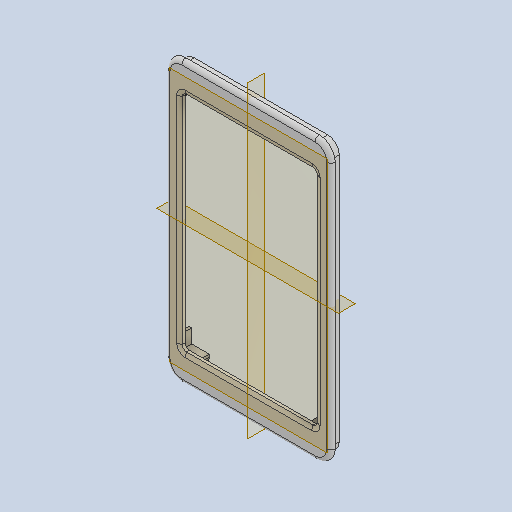
# Autodesk Inventor part: front-bezel
Saved by Autodesk Inventor 2024 (Build 280153000, 153)
## iProperties
Created: 2024-08-25
Part Number: front-bezel
Material: Generic
Document SubType Name: Modeling
Designer: Stefano
Density: 1 g/cm^3
Appearance: Default
Author: Stefano
Autodesk Inventor part; units mm, degrees
ref_plane "YZ Plane" through (0, 0, 0) normal (1, 0, 0) x (0, 1, 0)
ref_plane "Work Plane1" through (0, 0, 2.9972) normal (0, 0, 1) x (1, 0, 0)
ref_plane "Work Plane3" through (-58.9, -99.9, 0) normal (0, 0, 1) x (1, 0, 0)
sketch "Sketch2" plane through (0, 0, 2.9972) normal (0, 0, 1) x (1, 0, 0)
  line L0 (51.1175, 82.55) -> (51.1175, -82.55) construction
  line L1 (-51.1175, 82.55) -> (51.1175, 82.55) construction
  line L2 (-51.1175, -82.55) -> (-51.1175, 82.55) construction
  line L3 (51.1175, -82.55) -> (-51.1175, -82.55) construction
  arc A0 (58.9, 88.5) -> (47.5, 99.9) centre (47.5, 88.5) ccw projected
  line L4 (47.5, 99.9) -> (-47.5, 99.9) projected
  line L5 (58.9, -88.5) -> (58.9, 88.5) projected
  arc A1 (47.5, -99.9) -> (58.9, -88.5) centre (47.5, -88.5) ccw projected
  line L6 (-47.5, -99.9) -> (47.5, -99.9) projected
  arc A2 (-58.9, -88.5) -> (-47.5, -99.9) centre (-47.5, -88.5) ccw projected
  line L7 (-58.9, 88.5) -> (-58.9, -88.5) projected
  arc A3 (-47.5, 99.9) -> (-58.9, 88.5) centre (-47.5, 88.5) ccw projected
  line L8 (48.1175, -79.55) -> (48.1175, 79.55)
  line L9 (48.1175, 79.55) -> (-48.1175, 79.55)
  line L10 (-48.1175, 79.55) -> (-48.1175, -79.55)
  line L11 (-48.1175, -79.55) -> (48.1175, -79.55)
  point P0 (0, 0)
  dimension "d1" = 3
  constraints: 8 end point, 3 other
  measures "d1" distance between parallel lines of L0 L8
extrude "Extrusion1" add sketch "Sketch2" against normal up to surface (2.9972 mm away)
fillet "Fillet1" radius 3 4 edges at (48.1175, 79.55, 1.4986) (48.1175, -79.55, 1.4986) (-48.1175, -79.55, 1.4986) (-48.1175, 79.55, 1.4986)
chamfer "Chamfer1" distance 3 distance2 1 4 edges at (48.1175, 0, 2.9972) (0, -79.55, 2.9972) (-48.1175, 0, 2.9972) (0, 79.55, 2.9972) measured on face at (15.0392, -93.1167, 2.9972)
sketch "Sketch3" plane through (47.5, 99.9, 0) normal (0, 0, -1) x (-1, 0, 0)
  line L0 (98.6175, -17.35) -> (-3.6175, -17.35) construction
  line L1 (98.6175, -182.45) -> (98.6175, -17.35) construction
  line L2 (-3.6175, -182.45) -> (98.6175, -182.45) construction
  line L3 (-3.6175, -17.35) -> (-3.6175, -182.45) construction
  line L4 (95, -196.8) -> (0, -196.8) construction
  arc A0 (-8.4, -188.4) -> (0, -196.8) centre (0, -188.4) ccw construction
  line L5 (-8.4, -188.4) -> (-8.4, -11.4) construction
  arc A1 (0, -3) -> (-8.4, -11.4) centre (0, -11.4) ccw construction
  line L6 (0, -3) -> (95, -3) construction
  arc A2 (103.4, -11.4) -> (95, -3) centre (95, -11.4) ccw construction
  line L7 (103.4, -11.4) -> (103.4, -188.4) construction
  arc A3 (95, -196.8) -> (103.4, -188.4) centre (95, -188.4) ccw construction
  line L8 (-3.7175, -17.25) -> (98.7175, -17.25)
  line L9 (98.7175, -17.25) -> (98.7175, -182.55)
  line L10 (98.7175, -182.55) -> (-3.7175, -182.55)
  line L11 (-3.7175, -182.55) -> (-3.7175, -17.25)
  line L12 (95, -3.1) -> (0, -3.1)
  arc A4 (0, -3.1) -> (-8.3, -11.4) centre (0, -11.4) ccw
  line L13 (-8.3, -11.4) -> (-8.3, -188.4)
  arc A5 (-8.3, -188.4) -> (0, -196.7) centre (0, -188.4) ccw
  line L14 (0, -196.7) -> (95, -196.7)
  arc A6 (95, -196.7) -> (103.3, -188.4) centre (95, -188.4) ccw
  line L15 (103.3, -188.4) -> (103.3, -11.4)
  arc A7 (103.3, -11.4) -> (95, -3.1) centre (95, -11.4) ccw
  line L16 (100.7175, -15.25) -> (-5.7175, -15.25)
  line L17 (-5.7175, -15.25) -> (-5.7175, -184.55)
  line L18 (-5.7175, -184.55) -> (100.7175, -184.55)
  line L19 (100.7175, -184.55) -> (100.7175, -15.25)
  line L20 (100.7175, -172.55) -> (98.7175, -172.55)
  arc A8 (86.2825, -184.55) -> (100.7175, -184.55) centre (93.5, -184.55) ccw
  line L21 (86.2825, -184.55) -> (86.2825, -182.55)
  circle A9 centre (93.5, -177.4) radius 1.0065 construction
  line L22 (93.5, -177.4) -> (93.5, -184.55) construction
  point P0 (47.5, -99.9)
  dimension "d8" = 0.1
  dimension "d9" = 0.1
  dimension "d10" = 2
  dimension "d11" = 12
  constraints: 30 end point, 10 point on circle, 5 centre point, 4 point on line, 3 perpendicular, 2 tangent, 13 other
  measures "d8" distance between parallel lines of L0 L8
  measures "d9" radial gap between concentric circles of A2 A7
  measures "d10" distance between parallel lines of L8 L16
  measures "d11" distance between parallel lines of L18 L20
ref_plane "Work Plane4" through (-51.1175, -82.55, -7.874) normal (0, 0, -1) x (0, 1, 0)
extrude "Extrusion2" add sketch "Sketch3" along normal up to surface (7.874 mm away) contours L20 L19 L18 L21 L10 L9 | L18 A8
ref_plane "Work Plane5" through (0, -88.5, 2.9972) normal (1, 0, 0) x (0, 0, -1)
ref_plane "Work Plane6" through (-47.5, 0, 2.9972) normal (0, 1, 0) x (1, 0, 0)
sketch "Sketch5" plane through (-46, -84.65, -7.874) normal (0, 0, -1) x (-1, 0, 0)
  arc A0 (-7.2175, 0) -> (7.2175, 0) centre (0, 0) ccw projected
  line L0 (0, -7.2175) -> (0, 2) construction
  line L1 (-7.2175, 2) -> (5.2175, 2) projected
  point P0 (-46, 84.65)
  point P1 (0, -2.6087)
  constraints: 2 end point, 2 midpoint, 2 point on line, 1 point on circle, 1 vertical
hole "Hole1" at (-46, -87.2587, -7.874) direction (0, 0, 1) diameter 3 depth 6 tip angle 118
mirror "Mirror1" about plane through (0, -88.5, 2.9972) normal (1, 0, 0) of "Extrusion2", "Hole1"
mirror "Mirror2" about plane through (-47.5, 0, 2.9972) normal (0, 1, 0) of "Extrusion2", "Hole1", "Mirror1"
fillet "Fillet2" radius 3 8 edges at (55.561, -96.561, 2.9972) (58.9, 0, 2.9972) (55.561, 96.561, 2.9972) (0, 99.9, 2.9972) (-55.561, 96.561, 2.9972) (-58.9, 0, 2.9972) (-55.561, -96.561, 2.9972) (0, -99.9, 2.9972)
sketch "Sketch6" plane through (47.5, 99.9, 0) normal (0, 0, -1) x (-1, 0, 0)
  line L0 (95, -196.8) -> (0, -196.8) construction
  line L1 (-8.4, -188.4) -> (-8.4, -11.4) construction
  line L2 (0, -3) -> (95, -3) construction
  line L3 (103.4, -11.4) -> (103.4, -188.4) construction
  arc A0 (-8.4, -188.4) -> (0, -196.8) centre (0, -188.4) ccw construction
  arc A1 (0, -3) -> (-8.4, -11.4) centre (0, -11.4) ccw construction
  arc A2 (103.4, -11.4) -> (95, -3) centre (95, -11.4) ccw construction
  arc A3 (95, -196.8) -> (103.4, -188.4) centre (95, -188.4) ccw construction
  line L4 (0, -196.7) -> (95, -196.7)
  arc A4 (95, -196.7) -> (103.3, -188.4) centre (95, -188.4) ccw
  line L5 (103.3, -188.4) -> (103.3, -11.4)
  arc A5 (103.3, -11.4) -> (95, -3.1) centre (95, -11.4) ccw
  line L6 (95, -3.1) -> (0, -3.1)
  arc A6 (0, -3.1) -> (-8.3, -11.4) centre (0, -11.4) ccw
  line L7 (-8.3, -11.4) -> (-8.3, -188.4)
  arc A7 (-8.3, -188.4) -> (0, -196.7) centre (0, -188.4) ccw
  line L8 (-7.3, -188.4) -> (-7.3, -11.4)
  arc A8 (0, -4.1) -> (-7.3, -11.4) centre (0, -11.4) ccw
  line L9 (0, -4.1) -> (95, -4.1)
  arc A9 (102.3, -11.4) -> (95, -4.1) centre (95, -11.4) ccw
  line L10 (102.3, -11.4) -> (102.3, -188.4)
  arc A10 (95, -195.7) -> (102.3, -188.4) centre (95, -188.4) ccw
  line L11 (95, -195.7) -> (0, -195.7)
  arc A11 (-7.3, -188.4) -> (0, -195.7) centre (0, -188.4) ccw
  arc A12 (23.5, -195.7) -> (11.5, -195.7) centre (17.5, -195.7) ccw
  line L12 (47.5, -195.7) -> (47.5, -4.1) construction
  arc A13 (83.5, -195.7) -> (71.5, -195.7) centre (77.5, -195.7) ccw
  line L13 (-7.3, -99.9) -> (102.3, -99.9) construction
  arc A14 (11.5, -4.1) -> (23.5, -4.1) centre (17.5, -4.1) ccw
  arc A15 (71.5, -4.1) -> (83.5, -4.1) centre (77.5, -4.1) ccw
  point P0 (47.5, -99.9)
  point P1 (11.5, -4.1)
  point P2 (23.5, -4.1)
  point P3 (83.5, -4.1)
  point P4 (83.5, -195.7)
  point P5 (71.5, -195.7)
  dimension "d22" = 0.1
  dimension "d23" = 1
  dimension "d24" = 6
  dimension "d34" = 60
  constraints: 24 point on circle, 20 end point, 12 centre point, 9 symmetric about line, 4 midpoint, 3 point on line, 17 other
  measures "d22" distance between parallel lines of L0 L4
  measures "d23" distance between parallel lines of L4 L11
  measures "d24" radius of A12
  measures "d34" distance of A13.centre A12.centre
extrude "Extrusion3" add sketch "Sketch6" along normal blind 6 contours A7 L7 A6 L6 A5 L5 A4 L4 | A12 L11 | L9 A14 | A13 L11 | L9 A15
sketch "Sketch8" plane through (47.5, 99.9, -6) normal (0, 0, -1) x (-1, 0, 0)
  line L0 (77.5, -6.1) -> (17.5, -6.1) construction
  line L1 (17.5, -6.1) -> (17.5, -193.7) construction
  line L2 (17.5, -193.7) -> (77.5, -193.7) construction
  line L3 (77.5, -193.7) -> (77.5, -6.1) construction
  line L4 (77.5, -6.1) -> (17.5, -193.7) construction
  line L5 (17.5, -6.1) -> (77.5, -193.7) construction
  line L6 (0, -196.7) -> (95, -196.7) construction
  point P0 (47.5, -99.9)
  dimension "d35" = 3
  dimension "d36" = 60
  constraints: 12 end point, 4 coincident, 2 midpoint, 2 parallel, 1 horizontal, 1 perpendicular
  measures "d35" distance from line of L6 L1.end
  measures "d36" distance between parallel lines of L1 L3
hole "Hole3" at (30, -93.8, -6) at (-30, -93.8, -6) at (-30, 93.8, -6) at (30, 93.8, -6) direction (0, 0, 1) diameter 3 depth 6 tip angle 118
body "Solid1"
